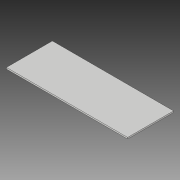
# Autodesk Inventor part: PowerSupplyEncSides
Saved by Autodesk Inventor 2019 (Build 230136000, 136)
## iProperties
Created: 2021-08-16
Part Number: PowerSupplyEncSides
Material: Generic
Document SubType Name: Modeling
Designer: devon
Density: 1 g/cm^3
Appearance: Default
Author: devon
Autodesk Inventor part; units mm, degrees
ref_plane "YZ Plane" through (0, 0, 0) normal (1, 0, 0) x (0, 1, 0)
ref_plane "XZ Plane" through (0, 0, 0) normal (0, 1, 0) x (-1, 0, 0)
ref_plane "XY Plane" through (0, 0, 0) normal (0, 0, 1) x (1, 0, 0)
sketch "Sketch1" plane through (0, 0, 0) normal (0, 1, 0) x (-1, 0, 0)
  line L0 (209.55, 79.375) -> (-209.55, 79.375)
  line L1 (-209.55, 79.375) -> (-209.55, -79.375)
  line L2 (-209.55, -79.375) -> (209.55, -79.375)
  line L3 (209.55, -79.375) -> (209.55, 79.375)
  line L4 (209.55, 79.375) -> (-209.55, -79.375) construction
  line L5 (-209.55, 79.375) -> (209.55, -79.375) construction
  point P0 (0, 0)
  dimension "d0" = 419.1
  dimension "d1" = 158.75
  constraints: 12 end point, 2 midpoint, 2 parallel, 1 horizontal, 1 perpendicular
  measures "d0" distance of L1.end L2.end
  measures "d1" distance of L2.end L0.start
extrude "Extrusion1" add sketch "Sketch1" along normal blind 5
body "Solid1"
